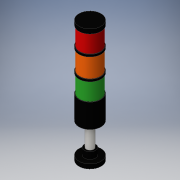
# Autodesk Inventor part: TowerLight
Saved by Autodesk Inventor 2016 (Build 200138000, 138)
## iProperties
Created: 2017-01-21
Part Number: TowerLight
Material: Generic
Document SubType Name: Modeling
Designer: Owner
Density: 1 g/cm^3
Appearance: Default
Author: Owner
Autodesk Inventor part; units mm, degrees
ref_plane "YZ Plane" through (0, 0, 0) normal (1, 0, 0) x (0, 1, 0)
ref_plane "XZ Plane" through (0, 0, 0) normal (0, 1, 0) x (-1, 0, 0)
ref_plane "XY Plane" through (0, 0, 0) normal (0, 0, 1) x (1, 0, 0)
sketch "Sketch1" plane through (0, 0, 0) normal (0, 1, 0) x (-1, 0, 0)
  line L0 (0, -35.56) -> (0, 35.56) projected
  line L1 (-35.56, 0) -> (35.56, 0) projected
  circle A0 centre (0, 0) radius 25.4
  dimension "d0" = 50.8
  constraints: 1 centre point, 1 coincident
  measures "d0" diameter of A0
extrude "Extrusion1" add sketch "Sketch1" along normal blind 279.4
sketch "Sketch2" plane through (0, 0, 0) normal (1, 0, 0) x (0, 1, 0)
  line L0 (279.4, -25.4) -> (279.4, 25.4) projected
  line L1 (0, 25.4) -> (0, -25.4) projected
  line L2 (0, -25.4) -> (279.4, -25.4) projected
  line L3 (0, 25.4) -> (10.16, 25.4)
  line L4 (10.16, 25.4) -> (10.16, -25.4)
  line L5 (10.16, -25.4) -> (0, -25.4)
  line L6 (0, -25.4) -> (0, 25.4)
  line L7 (-5.08, 12.7) -> (25.4, 12.7)
  line L8 (25.4, 12.7) -> (25.4, -12.7)
  line L9 (25.4, -12.7) -> (-5.08, -12.7)
  line L10 (-5.08, -12.7) -> (-5.08, 12.7)
  line L11 (-5.08, 12.7) -> (25.4, -12.7) construction
  line L12 (25.4, 12.7) -> (-5.08, -12.7) construction
  line L13 (-27.94, 8.6578) -> (78.74, 8.6578)
  line L14 (78.74, 8.6578) -> (78.74, -8.6578)
  line L15 (78.74, -8.6578) -> (-27.94, -8.6578)
  line L16 (-27.94, -8.6578) -> (-27.94, 8.6578)
  line L17 (-27.94, 8.6578) -> (78.74, -8.6578) construction
  line L18 (78.74, 8.6578) -> (-27.94, -8.6578) construction
  line L19 (78.74, 25.4) -> (0, 25.4)
  line L20 (0, 25.4) -> (0, -25.4)
  line L21 (0, -25.4) -> (78.74, -25.4)
  line L22 (78.74, -25.4) -> (78.74, 25.4)
  line L23 (25.4, 8.6578) -> (78.74, 8.6578)
  line L24 (78.74, 8.6578) -> (78.74, 25.4)
  line L25 (78.74, 25.4) -> (25.4, 25.4)
  line L26 (25.4, 25.4) -> (25.4, 8.6578)
  line L27 (10.16, 12.7) -> (25.4, 12.7)
  line L28 (25.4, 12.7) -> (25.4, 25.4)
  line L29 (25.4, 25.4) -> (10.16, 25.4)
  line L30 (10.16, 25.4) -> (10.16, 12.7)
  line L31 (10.16, -12.7) -> (25.4, -12.7)
  line L32 (25.4, -12.7) -> (25.4, -25.4)
  line L33 (25.4, -25.4) -> (10.16, -25.4)
  line L34 (10.16, -25.4) -> (10.16, -12.7)
  line L35 (25.4, -8.6578) -> (78.74, -8.6578)
  line L36 (78.74, -8.6578) -> (78.74, -25.4)
  line L37 (78.74, -25.4) -> (25.4, -25.4)
  line L38 (25.4, -25.4) -> (25.4, -8.6578)
  line L39 (-89.408, 0) -> (340.868, 0) projected
  point P0 (0, 0)
  point P1 (10.16, 0)
  point P2 (25.4, 0)
  dimension "d3" = 10.16
  dimension "d4" = 30.48
  dimension "d5" = 25.4
  dimension "d6" = 106.68
  constraints: 72 end point, 16 parallel, 10 midpoint, 8 horizontal, 8 perpendicular, 4 point on line
  measures "d3" distance of L4.end L5.end
  measures "d4" distance of L8.end L9.end
  measures "d5" distance of L7.end L8.end
  measures "d6" distance of L14.end L15.end
revolve "Revolution1" cut sketch "Sketch2" angle 360 about axis through (0, -10, 0) along (0, 1, 0) contours L2 L32 L8 L15 L22 | L2 L4 L9 L32 | L13 L8 L26 L19 L22 | L7 L4 L19 L26
sketch "Sketch3" plane through (0, 0, 0) normal (0, 0, 1) x (1, 0, 0)
  line L0 (25.4, 78.74) -> (-25.4, 78.74) projected
  line L1 (25.4, 78.74) -> (-25.4, 78.74) projected
  line L2 (25.4, 279.4) -> (-25.4, 279.4) projected
  line L3 (-25.4, 78.74) -> (25.4, 78.74)
  line L4 (25.4, 78.74) -> (25.4, 279.4)
  line L5 (25.4, 279.4) -> (-25.4, 279.4)
  line L6 (-25.4, 279.4) -> (-25.4, 78.74)
  line L7 (-25.4, 78.74) -> (-25.4, 279.4) projected
  line L8 (25.4, 279.4) -> (-25.4, 279.4)
  line L9 (-25.4, 279.4) -> (-25.4, 269.24)
  line L10 (-25.4, 269.24) -> (25.4, 269.24)
  line L11 (25.4, 269.24) -> (25.4, 279.4)
  line L12 (25.4, 78.74) -> (25.4, 279.4) projected
  line L13 (-25.4, 269.24) -> (25.4, 269.24)
  line L14 (25.4, 269.24) -> (25.4, 228.6)
  line L15 (25.4, 228.6) -> (-25.4, 228.6)
  line L16 (-25.4, 228.6) -> (-25.4, 269.24)
  line L17 (25.4, 228.6) -> (-25.4, 228.6)
  line L18 (-25.4, 228.6) -> (-25.4, 223.52)
  line L19 (-25.4, 223.52) -> (25.4, 223.52)
  line L20 (25.4, 223.52) -> (25.4, 228.6)
  line L21 (-25.4, 223.52) -> (15.24, 223.52)
  line L22 (15.24, 223.52) -> (15.24, 179.07)
  line L23 (15.24, 179.07) -> (-25.4, 179.07)
  line L24 (-25.4, 179.07) -> (-25.4, 223.52)
  line L25 (25.4, 179.07) -> (-25.4, 179.07)
  line L26 (-25.4, 179.07) -> (-25.4, 173.99)
  line L27 (-25.4, 173.99) -> (25.4, 173.99)
  line L28 (25.4, 173.99) -> (25.4, 179.07)
  line L29 (-25.4, 173.99) -> (25.4, 173.99)
  line L30 (25.4, 173.99) -> (25.4, 133.35)
  line L31 (25.4, 133.35) -> (-25.4, 133.35)
  line L32 (-25.4, 133.35) -> (-25.4, 173.99)
  line L33 (0, 269.24) -> (-24.13, 269.24)
  line L34 (-24.13, 269.24) -> (-24.13, 228.6)
  line L35 (-24.13, 228.6) -> (0, 228.6)
  line L36 (0, 228.6) -> (0, 269.24)
  line L37 (-25.4, 228.6) -> (-24.13, 228.6)
  line L38 (-24.13, 228.6) -> (-24.13, 269.24)
  line L39 (-24.13, 269.24) -> (-25.4, 269.24)
  line L40 (-25.4, 269.24) -> (-25.4, 228.6)
  line L41 (-25.4, 179.07) -> (-24.13, 179.07)
  line L42 (-24.13, 179.07) -> (-24.13, 223.52)
  line L43 (-24.13, 223.52) -> (-25.4, 223.52)
  line L44 (-25.4, 223.52) -> (-25.4, 179.07)
  line L45 (-25.4, 173.99) -> (-24.13, 173.99)
  line L46 (-24.13, 173.99) -> (-24.13, 133.35)
  line L47 (-24.13, 133.35) -> (-25.4, 133.35)
  line L48 (-25.4, 133.35) -> (-25.4, 173.99)
  point P0 (0, 0)
  dimension "d8" = 10.16
  dimension "d9" = 40.64
  dimension "d10" = 5.08
  dimension "d11" = 40.64
  dimension "d12" = 5.08
  dimension "d13" = 40.64
  dimension "d14" = 24.13
  dimension "d15" = 1.27
  dimension "d16" = 1.27
  dimension "d17" = 40.64
  constraints: 88 end point, 22 parallel, 11 horizontal, 11 perpendicular, 7 point on line, 2 midpoint
  measures "d8" distance of L9.end L8.end
  measures "d9" distance of L13.end L14.end
  measures "d10" distance of L18.end L17.end
  measures "d11" distance of L22.end L23.end
  measures "d12" distance of L26.end L25.end
  measures "d13" distance of L29.end L30.end
  measures "d14" distance of L35.end L34.end
  measures "d15" distance of L43.end L42.end
  measures "d16" distance of L46.end L47.end
  measures "d17" distance of L45.end L46.end
revolve "Revolution2" cut sketch "Sketch3" angle 360 about axis through (0, 228.6, 0) along (0, 1, 0) contours L6 L27 L46 L31 | L6 L19 L42 L23 | L6 L10 L34 L15
body "Solid1"
